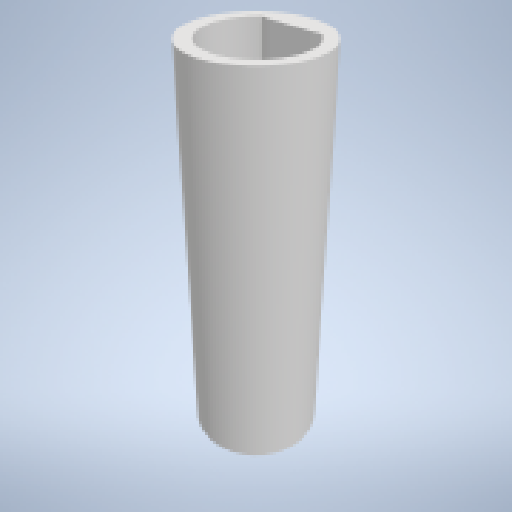
# Autodesk Inventor part: acoplador
Saved by Autodesk Inventor 2023 (Build 270158000, 158)
## iProperties
Created: 2022-10-13
Part Number: acoplador
Material: Generic
Document SubType Name: Modeling
Designer: klebe
Density: 1 g/cm^3
Appearance: Default
Description: Acoplador motor
Author: klebe
Autodesk Inventor part; units mm, degrees
note: some values were not read from the file. Chosen so that the rebuilt part matches the saved one: second side of "Extrusion1".
ref_plane "YZ Plane" through (0, 0, 0) normal (1, 0, 0) x (0, 1, 0)
ref_plane "XZ Plane" through (0, 0, 0) normal (0, 1, 0) x (-1, 0, 0)
ref_plane "XY Plane" through (0, 0, 0) normal (0, 0, 1) x (1, 0, 0)
sketch "Sketch1" plane through (0, 0, 0) normal (0, 1, 0) x (-1, 0, 0)
  circle A0 centre (66.0648, 12.7211) radius 2.5 projected
  circle A1 centre (66.0648, 12.7211) radius 2.5
  point P0 (0, 0)
  dimension "d7" = 5
  constraints: 1 centre point, 1 coincident
  measures "d7" diameter of A1
extrude "Extrusion1" add sketch "Sketch1" along normal blind 16
sketch "Sketch2" plane through (-66.0648, 16, 12.7211) normal (0, 1, 0) x (1, 0, 0)
  line L0 (0.8397, 1.4867) -> (-0.9155, 1.4912)
  ellipse E0 centre (0.0567, 0.0303) end of major axis (-0.8862, 1.7941) minor radius 1.9327 (-1.2692, 1.5225) -> (1.3068, 1.516) ccw
  spline S0 degree 2 poles (1.3068, 1.516) (1.0542, 1.4985) (0.8397, 1.4867) knots 0 0 0 1 1 1 weights 1 1.006377 1
  spline S1 degree 2 poles (-0.9155, 1.4912) (-1.084, 1.5039) (-1.2692, 1.5225) knots 0 0 0 1 1 1 weights 1 1.006377 1
  point P0 (66.0648, 12.7211)
  point P1 (-1.3518, 1.4745)
  constraints: 1 other
extrude "Extrusion5" cut sketch "Sketch2" against normal blind 9
body "Solid1"
